Autodesk Inventor part; units mm, degrees
(part 2 of 2)
sketch "Sketch24" plane through (0, 0, 2.4) normal (0, 0, 1) x (1, 0, 0)
  circle A0 centre (-21.5, -6.85) radius 1.5 projected
  circle A1 centre (21.5, -6.85) radius 1.5 projected
  line L0 (7, 28.1737) -> (7, 22.8553) projected
  line L1 (7, 22.8553) -> (-7, 22.8553) projected
  line L2 (-7, 22.8553) -> (-7, 28.1737) projected
  line L3 (-7, 28.1737) -> (-28, 28.1737) projected
  line L4 (-28, 28.1737) -> (-28, 36.1074) projected
  line L5 (-28, 36.1074) -> (-41, 36.1074) projected
  line L6 (-41, 36.1074) -> (-41, 28.0794) projected
  line L7 (-41, 28.0794) -> (-35, 28.0794) projected
  line L8 (-35, 28.0794) -> (-35, 17.0794) projected
  line L9 (-35, 17.0794) -> (-41, 17.0794) projected
  line L10 (-41, 17.0794) -> (-41, -14.85) projected
  line L11 (-41, -14.85) -> (-18, -14.85) projected
  line L12 (-18, -14.85) -> (-18, -1.85) projected
  line L13 (-18, -1.85) -> (-2.5, -1.85) projected
  line L14 (-2.5, -1.85) -> (-2.5, -46.05) projected
  line L15 (-2.5, -46.05) -> (2.5, -46.05) projected
  line L16 (2.5, -46.05) -> (2.5, -1.85) projected
  line L17 (2.5, -1.85) -> (18, -1.85) projected
  line L18 (18, -1.85) -> (18, -14.85) projected
  line L19 (18, -14.85) -> (41, -14.85) projected
  line L20 (41, -14.85) -> (41, 17.0794) projected
  line L21 (41, 17.0794) -> (35.2556, 17.0794) projected
  line L22 (35.2556, 17.0794) -> (35.2556, 28.0794) projected
  line L23 (35.2556, 28.0794) -> (41, 28.0794) projected
  line L24 (41, 28.0794) -> (41, 36.1074) projected
  line L25 (41, 36.1074) -> (28, 36.1074) projected
  line L26 (28, 36.1074) -> (28, 28.1737) projected
  line L27 (28, 28.1737) -> (7, 28.1737) projected
  line L28 (-7, 22.8553) -> (7, 22.8553) projected
  line L29 (7, 22.8553) -> (7, 28.1737) projected
  line L30 (7, 28.1737) -> (-7, 28.1737) projected
  line L31 (-7, 28.1737) -> (-7, 22.8553) projected
  line L32 (15.8857, 14.0076) -> (5.4393, 16.3235)
  line L33 (5.7856, 17.8856) -> (5.4393, 16.3235)
  line L34 (5.7856, 17.8856) -> (16.232, 15.5697)
  line L35 (16.232, 15.5697) -> (15.8857, 14.0076)
  line L36 (-1.5875, 18.8163) -> (-1.2412, 17.2542)
  line L37 (-12.0339, 16.5004) -> (-1.5875, 18.8163)
  line L38 (-1.2412, 17.2542) -> (-11.6876, 14.9383)
  line L39 (-12.0339, 16.5004) -> (-11.6876, 14.9383)
  line L40 (-36.4173, 12.4288) -> (-35.4433, 11.1595)
  line L41 (-36.4173, 12.4288) -> (-27.9284, 18.9426)
  line L42 (-26.9544, 17.6732) -> (-35.4433, 11.1595)
  line L43 (-27.9284, 18.9426) -> (-26.9544, 17.6732)
  line L44 (-32.1332, 15.7161) -> (-32.8028, 16.5888)
  line L45 (-35.6239, 13.0376) -> (-36.2936, 13.9103)
  line L46 (-30.9981, 0.0141) -> (-35.9388, -9.4769)
  line L47 (-32.4173, 0.7529) -> (-30.9981, 0.0141)
  line L48 (-37.358, -8.7381) -> (-32.4173, 0.7529)
  line L49 (-37.358, -8.7381) -> (-35.9388, -9.4769)
  line L50 (31.3398, 16.3249) -> (30.3658, 15.0555)
  line L51 (31.3398, 16.3249) -> (39.8287, 9.8111)
  line L52 (38.8547, 8.5418) -> (30.3658, 15.0555)
  line L53 (39.8287, 9.8111) -> (38.8547, 8.5418)
  line L54 (34.4028, -3.0613) -> (32.9836, -3.8001)
  line L55 (34.4028, -3.0613) -> (39.3435, -12.5523)
  line L56 (37.9243, -13.2911) -> (32.9836, -3.8001)
  line L57 (39.3435, -12.5523) -> (37.9243, -13.2911)
  line L58 (-34.8646, -3.9483) -> (-35.8403, -3.4404)
  line L59 (-36.8963, -7.8511) -> (-37.872, -7.3432)
  line L60 (-11.0576, 16.7168) -> (-11.2957, 17.7907)
  line L61 (-6.7619, 17.6691) -> (-7, 18.7431)
  line L62 (6.7619, 17.6691) -> (7, 18.7431)
  line L63 (11.0576, 16.7168) -> (11.2957, 17.7907)
  line L64 (32.1332, 15.7161) -> (32.8028, 16.5888)
  line L65 (35.6239, 13.0376) -> (36.2936, 13.9103)
  line L66 (34.8646, -3.9483) -> (35.8403, -3.4404)
  line L67 (36.8963, -7.8511) -> (37.872, -7.3432)
  line L68 (37.872, -7.3432) -> (35.8403, -3.4404)
  line L69 (32.8028, 16.5888) -> (36.2936, 13.9103)
  line L70 (7, 18.7431) -> (11.2957, 17.7907)
  line L71 (-11.2957, 17.7907) -> (-7, 18.7431)
  line L72 (-36.2936, 13.9103) -> (-32.8028, 16.5888)
  line L73 (-37.872, -7.3432) -> (-35.8403, -3.4404)
  point P0 (0, 0)
  constraints: 84 end point, 1 parallel, 1 point on line, 84 other
extrude "Extrusion24" cut sketch "Sketch24" against normal through all contours L32 L33 L34 L35 | L34 L62 L70 L63 | L36 L38 L39 L37 | L37 L60 L71 L61 | L41 L43 L42 L40 | L45 L72 L44 L41 | L46 L49 L48 L47 | L48 L59 L73 L58 | L51 L53 L52 L50 | L64 L69 L65 L51 | L55 L57 L56 L54 | L66 L68 L67 L55
sketch "Sketch25" plane through (0, 0, 2.4) normal (0, 0, 1) x (1, 0, 0)
  line L0 (-7, 22.8553) -> (7, 22.8553) projected
  line L1 (7, 22.8553) -> (7, 28.1737) projected
  line L2 (7, 28.1737) -> (-7, 28.1737) projected
  line L3 (-7, 28.1737) -> (-7, 22.8553) projected
  point P0 (0, 0)
extrude "Extrusion25" cut sketch "Sketch25" along normal through all
body "Solid1"
